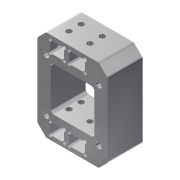
# Autodesk Inventor part: supportHolder
Saved by Autodesk Inventor 2015 (Build 190159000, 159)
## iProperties
Created: 2016-04-14
Part Number: supportHolder
Material: Generic
Document SubType Name: Modeling
Designer: jad211
Density: 1 g/cm^3
Appearance: Aluminum - Dark
Author: jad211
Autodesk Inventor part; units mm, degrees
ref_plane "YZ Plane" through (0, 0, 0) normal (1, 0, 0) x (0, 1, 0)
ref_plane "XZ Plane" through (0, 0, 0) normal (0, 1, 0) x (-1, 0, 0)
ref_plane "XY Plane" through (0, 0, 0) normal (0, 0, 1) x (1, 0, 0)
sketch "Sketch1" plane through (0, 0, 0) normal (0, 1, 0) x (-1, 0, 0)
  circle A0 centre (0, 0) radius 35
  circle A1 centre (15, 15) radius 1.6
  circle A2 centre (15, -15) radius 1.6
  circle A3 centre (-15, -15) radius 1.6
  circle A4 centre (-15, 15) radius 1.6
  line L0 (15, 15) -> (-15, 15) construction
  line L1 (-15, 15) -> (-15, -15) construction
  line L2 (-15, -15) -> (15, -15) construction
  line L3 (15, -15) -> (15, 15) construction
  circle A5 centre (0, 0) radius 10
  dimension "d1" = 30
  dimension "d2" = 30
  dimension "d4" = 3.2
  dimension "d5" = 3.2
  dimension "d6" = 3.2
  dimension "d7" = 3.2
  dimension "d8" = 15
  dimension "d9" = 15
  dimension "d10" = 20
  dimension "d11" = 70
  constraints: 8 end point, 6 centre point, 4 coincident, 2 parallel, 1 horizontal, 1 perpendicular
  measures "d1" distance of A2.centre L1.end
  measures "d2" distance of L0.start A2.centre
  measures "d4" diameter of A1
  measures "d5" diameter of A2
  measures "d6" diameter of A3
  measures "d7" diameter of A4
  measures "d8" distance from line of point (0, 0) L3
  measures "d9" horizontal distance of L1.end point (0, 0)
  measures "d10" diameter of A5
  measures "d11" diameter of A0
extrude "Extrusion1" add sketch "Sketch1" along normal blind 20
sketch "Sketch2" plane through (0, 20, 0) normal (0, 1, 0) x (1, 0, 0)
  circle A0 centre (-15, -15) radius 1.6 projected
  circle A1 centre (-15, -15) radius 2.5
  circle A2 centre (-15, 15) radius 1.6 projected
  circle A3 centre (-15, 15) radius 2.5
  circle A4 centre (15, 15) radius 2.5
  circle A5 centre (15, -15) radius 2.5
  point P0 (0, 0)
  dimension "d14" = 15
  dimension "d15" = 15
  dimension "d16" = 15
  dimension "d17" = 15
  dimension "d18" = 5
  dimension "d19" = 5
  dimension "d20" = 5
  dimension "d21" = 5
  constraints: 4 centre point, 2 coincident
  measures "d14" horizontal distance of point (0, 0) A4.centre
  measures "d15" horizontal distance of point (0, 0) A4.centre
  measures "d16" horizontal distance of point (0, 0) A5.centre
  measures "d17" horizontal distance of point (0, 0) A5.centre
  measures "d18" diameter of A1
  measures "d19" diameter of A3
  measures "d20" diameter of A5
  measures "d21" diameter of A4
extrude "Extrusion2" cut sketch "Sketch2" against normal blind 15
sketch "Sketch3" plane through (0, 20, 0) normal (0, 1, 0) x (1, 0, 0)
  line L0 (-12.75, -23.45) -> (-4.841, -23.45)
  line L1 (-4.841, -23.45) -> (-4.841, -17)
  line L2 (-4.841, -17) -> (-12.75, -17)
  line L3 (-12.75, -17) -> (-12.75, -23.45)
  line L4 (-1.941, -23.45) -> (7.059, -23.45)
  line L5 (7.059, -23.45) -> (7.059, -17)
  line L6 (7.059, -17) -> (-1.941, -17)
  line L7 (-1.941, -17) -> (-1.941, -23.45)
  line L8 (-11.75, 17) -> (-5.841, 17)
  line L9 (-4.841, 18) -> (-4.841, 22.3739)
  line L10 (-5.8263, 23.45) -> (-11.7381, 23.45)
  line L11 (-12.7499, 22.4501) -> (-12.7499, 18)
  line L12 (-0.941, 17) -> (6.059, 17)
  line L13 (7.059, 18) -> (7.059, 22.45)
  line L14 (6.059, 23.45) -> (-0.941, 23.45)
  line L15 (-1.941, 22.45) -> (-1.941, 18)
  arc A0 (-12.7499, 18) -> (-11.75, 17) centre (-12.75, 17) ccw
  arc A1 (-11.7381, 23.45) -> (-12.7499, 22.4501) centre (-12.7381, 23.45) ccw
  arc A2 (-4.841, 22.3739) -> (-5.8263, 23.45) centre (-4.8292, 23.3739) ccw
  arc A3 (-5.841, 17) -> (-4.841, 18) centre (-4.841, 17) ccw
  arc A4 (7.059, 22.45) -> (6.059, 23.45) centre (7.059, 23.45) ccw
  arc A5 (6.059, 17) -> (7.059, 18) centre (7.059, 17) ccw
  arc A6 (-1.941, 18) -> (-0.941, 17) centre (-1.941, 17) ccw
  arc A7 (-0.941, 23.45) -> (-1.941, 22.45) centre (-1.941, 23.45) ccw
  point P0 (0, 0)
  dimension "d24" = 17
  dimension "d25" = 17
  dimension "d26" = 6.45
  dimension "d27" = 6.45
  dimension "d28" = 2.9
  dimension "d29" = 7.909
  dimension "d30" = 9
  dimension "d31" = 1.941
  dimension "d32" = 34
  dimension "d33" = 6.45
  dimension "d42" = 2
  dimension "d43" = 2
  dimension "d44" = 2
  dimension "d45" = 2
  dimension "d46" = 2
  dimension "d47" = 2
  dimension "d50" = 2
  dimension "d51" = 2
  constraints: 32 end point, 16 point on circle, 8 centre point, 8 parallel, 4 horizontal, 4 perpendicular, 2 collinear
  measures "d24" distance from line of point (0, 0) L2
  measures "d25" distance from line of point (0, 0) L6
  measures "d26" distance of L2.end L0.start
  measures "d27" distance of L6.end L4.start
  measures "d28" distance between parallel lines of L7 L1
  measures "d29" distance of L0.start L0.end
  measures "d30" distance between parallel lines of L5 L7
  measures "d31" distance from line of point (0, 0) L7
  measures "d32" distance between parallel lines of L2 L8
  measures "d33" distance of L10.end L8.start
  measures "d42" diameter of A3
  measures "d43" diameter of A2
  measures "d44" diameter of A1
  measures "d45" diameter of A0
  measures "d46" diameter of A5
  measures "d47" diameter of A4
  measures "d50" diameter of A6
  measures "d51" diameter of A7
extrude "Extrusion3" cut sketch "Sketch3" against normal blind 25
sketch "Sketch5" plane through (0, 20, 0) normal (0, 1, 0) x (1, 0, 0)
  line L0 (-20, -26) -> (20, -26)
  line L1 (20, -26) -> (20, 26)
  line L2 (20, 26) -> (-20, 26)
  line L3 (-20, 26) -> (-20, -26)
  line L4 (-12.5, -12.5) -> (12.5, -12.5)
  line L5 (12.5, -12.5) -> (12.5, 12.5)
  line L6 (12.5, 12.5) -> (-12.5, 12.5)
  line L7 (-12.5, 12.5) -> (-12.5, -12.5)
  point P0 (0, 0)
  dimension "d64" = 52
  dimension "d65" = 40
  dimension "d66" = 20
  dimension "d67" = 26
  dimension "d70" = 25
  dimension "d71" = 25
  dimension "d72" = 12.5
  dimension "d73" = 12.5
  constraints: 16 end point, 4 parallel, 2 horizontal, 2 perpendicular
  measures "d64" distance of L2.end L0.start
  measures "d65" distance of L1.end L2.end
  measures "d66" distance from line of point (0, 0) L3
  measures "d67" distance from line of L2 point (0, 0)
  measures "d70" distance of L6.end L4.start
  measures "d71" distance of L5.end L6.end
  measures "d72" distance from line of point (0, 0) L7
  measures "d73" distance from line of L6 point (0, 0)
extrude "Extrusion5" cut sketch "Sketch5" against normal blind 30 keep common part
fillet "Fillet1" radius 2 1 edges at (-20, 10, 26)
fillet "Fillet2" radius 2 1 edges at (20, 10, 26)
fillet "Fillet3" radius 2 1 edges at (20, 10, -26)
fillet "Fillet4" radius 2 1 edges at (-20, 10, -26)
fillet "Fillet5" radius 2 1 edges at (12.5, 10, 12.5)
fillet "Fillet6" radius 2 1 edges at (-12.5, 10, -12.5)
fillet "Fillet7" radius 2 2 edges at (12.5, 10, -12.5) (-12.5, 10, 12.5)
sketch "Sketch6" plane through (-18, 0, 26) normal (0, 0, 1) x (1, 0, 0)
  circle A0 centre (9, 7) radius 1.55
  circle A1 centre (9, 14) radius 1.55
  circle A2 centre (21, 7) radius 1.55
  circle A3 centre (21, 14) radius 1.55
  line L0 (0, 0) -> (36, 0) projected
  line L1 (18, 0) -> (18, 20) construction
  dimension "d81" = 3.1
  dimension "d82" = 3.1
  dimension "d83" = 3.1
  dimension "d84" = 3.1
  dimension "d85" = 7
  dimension "d86" = 7
  dimension "d87" = 7
  dimension "d88" = 7
  dimension "d89" = 0
  dimension "d90" = 3
  dimension "d91" = 3
  dimension "d92" = 9
  dimension "d93" = 9
  constraints: 4 centre point, 2 end point, 1 midpoint, 1 vertical
  measures "d81" diameter of A1
  measures "d82" diameter of A0
  measures "d83" diameter of A2
  measures "d84" diameter of A3
  measures "d85" distance of A1.centre A0.centre
  measures "d86" distance from line of L0 A0.centre
  measures "d87" distance of A2.centre A3.centre
  measures "d88" distance from line of L0 A2.centre
  measures "d89" distance from line of point (18, 0) L1
  measures "d90" distance from line of L1 A3.centre
  measures "d91" distance from line of L1 A2.centre
  measures "d92" distance from line of L1 A1.centre
  measures "d93" distance from line of A0.centre L1
extrude "Extrusion6" cut sketch "Sketch6" against normal blind 100
sketch "Sketch7" plane through (0, 20, 0) normal (0, 1, 0) x (1, 0, 0)
  circle A0 centre (-15, -15) radius 2.5 projected
  circle A1 centre (-12.75, -23.45) radius 1
  circle A2 centre (-4.8235, -23.45) radius 1
  circle A3 centre (-4.841, -17) radius 1
  circle A4 centre (-1.941, -17) radius 1
  circle A5 centre (-1.941, -23.45) radius 1
  circle A6 centre (7.0924, -17) radius 1
  circle A7 centre (7.0924, -23.45) radius 1
  circle A8 centre (-12.75, -17) radius 1
  point P0 (0, 0)
  dimension "d96" = 2
  dimension "d97" = 2
  dimension "d98" = 2
  dimension "d99" = 2
  dimension "d100" = 2
  dimension "d101" = 2
  dimension "d102" = 2
  dimension "d103" = 2
  constraints: 8 centre point, 1 coincident
  measures "d96" diameter of A5
  measures "d97" diameter of A4
  measures "d98" diameter of A6
  measures "d99" diameter of A7
  measures "d100" diameter of A2
  measures "d101" diameter of A3
  measures "d102" diameter of A8
  measures "d103" diameter of A1
extrude "Extrusion7" cut sketch "Sketch7" against normal blind 100 contours A8 A0 | A0 A8 | A1 | A2 | A3 | A4 | A5 | A6 | A7 picked at (-13.2603, -16.5464) picked at (-12.7663, -16.994)
sketch "Sketch8" plane through (0, 0, 0) normal (0, -1, 0) x (1, 0, 0)
  line L0 (15, 26) -> (20, 21)
  line L1 (20, 24) -> (20, -24) projected
  line L2 (15, 26) -> (20, 26)
  line L3 (20, 21) -> (20, 26)
  line L4 (-18, 26) -> (18, 26) projected
  line L5 (-15, 26) -> (-20, 26)
  line L6 (-20, 26) -> (-20, 21)
  line L7 (-20, 21) -> (-15, 26)
  line L8 (-20, -24) -> (-20, 24) projected
  line L9 (-20, -21) -> (-20, -26)
  line L10 (-20, -26) -> (-15, -26)
  line L11 (-15, -26) -> (-20, -21)
  line L12 (18, -26) -> (-18, -26) projected
  line L13 (20, -21) -> (20, -26)
  line L14 (20, -26) -> (15, -26)
  line L15 (20, -21) -> (15, -26)
  point P0 (0, 0)
  dimension "d106" = 5
  dimension "d107" = 5
  dimension "d108" = 5
  dimension "d109" = 5
  dimension "d110" = 5
  dimension "d111" = 5
  dimension "d112" = 5
  dimension "d113" = 5
  constraints: 24 end point, 5 point on line, 3 perpendicular, 2 collinear, 2 horizontal, 2 vertical
  measures "d106" distance of L0.start L2.end
  measures "d107" distance of L0.end L2.end
  measures "d108" distance of L5.start L5.end
  measures "d109" distance of L5.end L6.end
  measures "d110" distance of L9.end L10.end
  measures "d111" distance of L9.start L9.end
  measures "d112" distance of L13.start L13.end
  measures "d113" distance of L13.end L14.end
extrude "Extrusion8" cut sketch "Sketch8" against normal blind 20 contours L2 L3 L1 L0 | L7 L6 L5 L4 | L1 L13 L14 L12 L15 | L11 L10 L9 L8
fillet "Fillet8" radius 2 1 edges at (15, 10, 26)
fillet "Fillet9" radius 2 1 edges at (20, 10, 21)
fillet "Fillet10" radius 2 1 edges at (20, 10, -21)
fillet "Fillet11" radius 2 3 edges at (15, 10, -26) (-15, 10, 26) (-20, 10, 21)
fillet "Fillet12" radius 2 2 edges at (-20, 10, -21) (-15, 10, -26)
equation "\"d5\" = d4"
equation "\"d6\" = d5"
equation "\"d7\" = d4"
equation "\"d19\" = d18"
equation "\"d20\" = d18"
equation "\"d21\" = d19"
equation "\"d25\" = d24"
equation "\"d27\" = d26"
equation "\"d32\" = 2 * d24"
equation "\"d33\" = d26"
equation "\"d66\" = 0.5 * d65"
equation "\"d67\" = 0.5 * d64"
equation "\"d72\" = 0.5 * d71"
equation "\"d87\" = d85"
equation "\"d88\" = d86"
body "Solid1"
